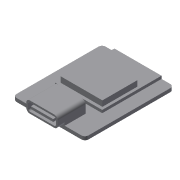
# Autodesk Inventor part: C3
Saved by Autodesk Inventor 2020 (Build 240168000, 168)
## iProperties
Created: 2022-10-11
Part Number: C3
Material: Allgemein
Document SubType Name: Modeling
Designer: uch10113
Density: 1 g/cm^3
Appearance: Vorgabe
Author: uch10113
Autodesk Inventor part; units mm, degrees
ref_plane "YZ Plane" through (0, 0, 0) normal (1, 0, 0) x (0, 1, 0)
ref_plane "XZ Plane" through (0, 0, 0) normal (0, 1, 0) x (-1, 0, 0)
ref_plane "XY Plane" through (0, 0, 0) normal (0, 0, 1) x (1, 0, 0)
sketch "Skizze1" plane through (0, 0, 0) normal (0, 0, 1) x (1, 0, 0)
  line L0 (-9.3, 12.75) -> (9.3, 12.75)
  line L1 (10.3, 11.75) -> (10.3, -11.75)
  line L2 (9.3, -12.75) -> (-9.3, -12.75)
  line L3 (-10.3, -11.75) -> (-10.3, 11.75)
  line L4 (-10.3, 12.75) -> (10.3, -12.75) construction
  line L5 (10.3, 12.75) -> (-10.3, -12.75) construction
  arc A0 (-9.3, 12.75) -> (-10.3, 11.75) centre (-9.3, 11.75) ccw
  arc A1 (10.3, 11.75) -> (9.3, 12.75) centre (9.3, 11.75) ccw
  arc A2 (9.3, -12.75) -> (10.3, -11.75) centre (9.3, -11.75) ccw
  arc A3 (-10.3, -11.75) -> (-9.3, -12.75) centre (-9.3, -11.75) ccw
  point P0 (0, 0)
  dimension "d0" = 20.6
  dimension "d1" = 25.5
  dimension "d2" = 1
  constraints: 12 end point, 8 point on circle, 8 point on line, 8 tangent, 4 centre point, 3 equal radius, 2 midpoint, 2 parallel, 1 horizontal, 1 perpendicular
  measures "d0" distance of L4.start L5.start
  measures "d1" distance of L5.end L4.start
  measures "d2" radius of A0
extrude "Extrusion1" add sketch "Skizze1" along normal blind 1
sketch "Skizze2" plane through (0, 0, 1) normal (0, 0, 1) x (1, 0, 0)
  line L0 (9.3, 12.75) -> (-9.3, 12.75) projected
  line L1 (-6.75, 12.75) -> (6.75, 12.75)
  line L2 (6.75, 12.75) -> (6.75, -4.25)
  line L3 (6.75, -4.25) -> (-6.75, -4.25)
  line L4 (-6.75, -4.25) -> (-6.75, 12.75)
  line L5 (-10.3, 11.75) -> (-10.3, -11.75) projected
  line L6 (10.3, -11.75) -> (10.3, 11.75) projected
  point P0 (0, 0)
  point P1 (6.75, 12.75)
  dimension "d5" = 13.5
  dimension "d6" = 3.55
  dimension "d7" = 3.55
  dimension "d8" = 17
  constraints: 8 end point, 2 parallel, 1 horizontal, 1 perpendicular, 1 point on line
  measures "d5" distance of L2.end L3.end
  measures "d6" distance between parallel lines of L5 L4
  measures "d7" distance between parallel lines of L2 L6
  measures "d8" distance of L1.end L2.end
extrude "Extrusion2" add sketch "Skizze2" along normal blind 0.8
sketch "Skizze3" plane through (0, 0, 1.8) normal (0, 0, 1) x (1, 0, 0)
  line L0 (6, -3.45) -> (-6, -3.45)
  line L1 (-6, -3.45) -> (-6, 6.55)
  line L2 (-6, 6.55) -> (6, 6.55)
  line L3 (6, 6.55) -> (6, -3.45)
  line L4 (-6.75, -4.25) -> (6.75, -4.25) projected
  point P0 (0, 0)
  dimension "d11" = 10
  dimension "d12" = 12
  dimension "d13" = 6
  dimension "d14" = 0.8
  constraints: 8 end point, 2 parallel, 1 horizontal, 1 perpendicular
  measures "d11" distance of L2.end L0.start
  measures "d12" distance of L1.end L2.end
  measures "d13" distance from line of point (0, 0) L1
  measures "d14" distance between parallel lines of L4 L0
extrude "Extrusion3" add sketch "Skizze3" along normal blind 1.6
sketch "Skizze4" plane through (0, 0, 1) normal (0, 0, 1) x (1, 0, 0)
  line L0 (4.5, -14.75) -> (-4.5, -14.75)
  line L1 (-4.5, -14.75) -> (-4.5, -6.75)
  line L2 (-4.5, -6.75) -> (4.5, -6.75)
  line L3 (4.5, -6.75) -> (4.5, -14.75)
  line L4 (-9.3, -12.75) -> (9.3, -12.75) projected
  point P0 (0, 0)
  dimension "d17" = 9
  dimension "d18" = 4.5
  dimension "d19" = 2
  dimension "d20" = 8
  constraints: 8 end point, 2 parallel, 1 horizontal, 1 perpendicular
  measures "d17" distance of L0.start L0.end
  measures "d18" distance from line of point (0, 0) L1
  measures "d19" distance between parallel lines of L4 L0
  measures "d20" distance of L2.end L0.start
extrude "Extrusion4" add sketch "Skizze4" along normal blind 3.3
fillet "Rundung1" radius 1 4 edges at (-4.5, -10.75, 4.3) (4.5, -10.75, 4.3) (-4.5, -13.75, 1) (4.5, -13.75, 1)
sketch "Skizze5" plane through (-3.5, -14.75, 1) normal (0, -1, 0) x (1, 0, 0)
  arc A0 (7, 0) -> (8, 1) centre (7, 1) ccw projected
  line L0 (8, 1) -> (8, 2.3) projected
  arc A1 (8, 2.3) -> (7, 3.3) centre (7, 2.3) ccw projected
  line L1 (0, 3.3) -> (7, 3.3) projected
  arc A2 (0, 3.3) -> (-1, 2.3) centre (0, 2.3) ccw projected
  line L2 (-1, 1) -> (-1, 2.3) projected
  arc A3 (-1, 1) -> (0, 0) centre (0, 1) ccw projected
  line L3 (0, 0) -> (7, 0) projected
  arc A4 (7.5, 2.3) -> (7, 2.8) centre (7, 2.3) ccw
  line L4 (7.5, 2.3) -> (7.5, 1)
  arc A5 (7, 0.5) -> (7.5, 1) centre (7, 1) ccw
  line L5 (7, 0.5) -> (0, 0.5)
  arc A6 (-0.5, 1) -> (0, 0.5) centre (0, 1) ccw
  line L6 (-0.5, 1) -> (-0.5, 2.3)
  arc A7 (0, 2.8) -> (-0.5, 2.3) centre (0, 2.3) ccw
  line L7 (0, 2.8) -> (7, 2.8)
  line L8 (6.7, 2) -> (6.7, 1.3)
  line L9 (6.7, 1.3) -> (0.3, 1.3)
  line L10 (0.3, 1.3) -> (0.3, 2)
  line L11 (0.3, 2) -> (6.7, 2)
  point P0 (3.5, -1)
  dimension "d24" = 0.5
  dimension "d25" = 0.8
  constraints: 16 end point, 8 point on circle, 4 centre point, 10 other
  measures "d24" distance between parallel lines of L1 L7
  measures "d25" distance between parallel lines of L7 L11
extrude "Extrusion5" cut sketch "Skizze5" against normal blind 3.3 contours L4 A5 L5 A6 L6 A7 L7 A4
sketch "Skizze6" plane through (0, 0, 0) normal (0, 0, -1) x (-1, 0, 0)
  line L0 (-6.8, 4.25) -> (6.8, 4.25)
  line L1 (6.8, 4.25) -> (6.8, -10.75)
  line L2 (6.8, -10.75) -> (-6.8, -10.75)
  line L3 (-6.8, -10.75) -> (-6.8, 4.25)
  line L4 (10.3, 11.75) -> (10.3, -11.75) projected
  line L5 (-10.3, -11.75) -> (-10.3, 11.75) projected
  line L6 (-9.3, 12.75) -> (9.3, 12.75) projected
  line L7 (9.3, -12.75) -> (-9.3, -12.75) projected
  point P0 (0, 0)
  dimension "d28" = 3.5
  dimension "d29" = 3.5
  dimension "d30" = 8.5
  dimension "d31" = 2
  constraints: 8 end point, 2 parallel, 1 horizontal, 1 perpendicular
  measures "d28" distance between parallel lines of L1 L4
  measures "d29" distance between parallel lines of L5 L3
  measures "d30" distance between parallel lines of L6 L0
  measures "d31" distance between parallel lines of L2 L7
extrude "Extrusion6" add sketch "Skizze6" along normal blind 0.8
equation "\"d6\" = d7"
equation "\"d13\" = 0.5 * d12"
equation "\"d18\" = 0.5 * d17"
equation "\"d29\" = d28"
